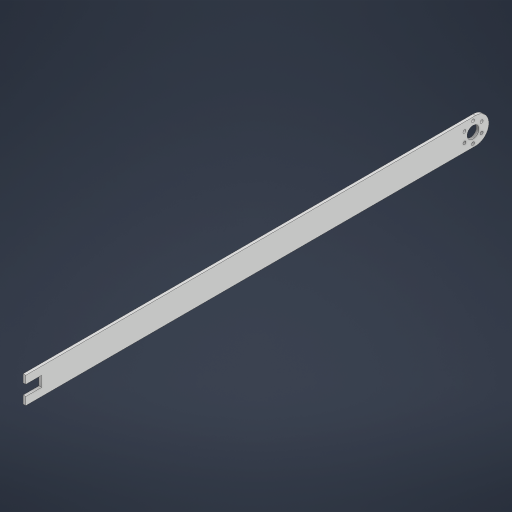
# Autodesk Inventor part: Arm
Saved by Autodesk Inventor 2023 (Build 270158000, 158)
## iProperties
Created: 2023-01-21
Part Number: Arm
Material: Generic
Document SubType Name: Modeling
Designer: Terrence
Density: 1 g/cm^3
Appearance: Default
Author: Terrence
Autodesk Inventor part; units mm, degrees
ref_plane "YZ Plane" through (0, 0, 0) normal (1, 0, 0) x (0, 1, 0)
ref_plane "XZ Plane" through (0, 0, 0) normal (0, 1, 0) x (-1, 0, 0)
ref_plane "XY Plane" through (0, 0, 0) normal (0, 0, 1) x (1, 0, 0)
sketch "Sketch1" plane through (0, 0, 0) normal (1, 0, 0) x (0, 1, 0)
  line L0 (0, -76.2) -> (63.5, -76.2)
  line L1 (63.5, -76.2) -> (63.5, -1193.8)
  line L2 (63.5, -1193.8) -> (0, -1193.8)
  line L3 (0, -1193.8) -> (0, -76.2)
  dimension "d0" = 63.5
  dimension "d1" = 1117.6
  constraints: 8 end point, 2 parallel, 1 horizontal, 1 perpendicular, 1 other
  measures "d0" distance of L1.end L2.end
  measures "d1" distance of L0.end L1.end
extrude "Extrusion1" add sketch "Sketch1" along normal blind 6.35
sketch "Sketch2" plane through (6.35, 0, 0) normal (1, 0, 0) x (0, 0, -1)
  line L0 (1193.8, 63.5) -> (76.2, 63.5) projected
  line L1 (1155.7, 63.5) -> (1155.7, 0) construction
  line L2 (0, 0) -> (1193.8, 0) projected
  circle A0 centre (1155.7, 31.75) radius 14.2875
  dimension "d5" = 1155.7
  dimension "d24" = 28.575
  constraints: 2 end point, 2 point on line, 1 centre point, 1 midpoint, 1 perpendicular
  measures "d5" distance from line of L2.start L1
  measures "d24" diameter of A0
extrude "Extrusion2" cut sketch "Sketch2" against normal through all
fillet "Fillet1" radius 31.75 2 edges at (3.175, 63.5, -1193.8) (3.175, 0, -1193.8)
sketch "Sketch5" plane through (6.35, 0, 0) normal (1, 0, 0) x (0, 0, -1)
  circle A0 centre (1155.7, 31.75) radius 14.2875 projected
  line L0 (1155.7, 31.75) -> (1155.7, 55.5752) construction
  circle A1 centre (1155.7, 55.5752) radius 3.6233
  point P0 (0, 0)
  dimension "d32" = 23.8252
  constraints: 2 end point, 1 centre point, 1 coincident, 1 vertical
  measures "d32" distance of L0.start L0.end
extrude "Extrusion5" cut sketch "Sketch5" against normal through all contours A1
pattern_circular "Circular Pattern1" count 6 over 360 about axis through (6.35, 31.75, -1155.7) along (-1, 0, 0) of "Extrusion5"
sketch "Sketch8" plane through (6.35, 0, 0) normal (1, 0, 0) x (0, 0, -1)
  line L0 (76.2, 44.45) -> (114.3, 44.45)
  line L1 (114.3, 44.45) -> (114.3, 19.05)
  line L2 (114.3, 19.05) -> (76.2, 19.05)
  line L3 (76.2, 19.05) -> (76.2, 44.45)
  line L4 (76.2, 63.5) -> (76.2, 0) projected
  point P0 (0, 0)
  point P1 (76.2, 31.75)
  dimension "d44" = 38.1
  dimension "d45" = 25.4
  constraints: 8 end point, 2 midpoint, 2 parallel, 1 horizontal, 1 perpendicular
  measures "d44" distance of L1.end L2.end
  measures "d45" distance of L2.end L0.start
extrude "Extrusion8" cut sketch "Sketch8" against normal blind 25.4
body "Solid1"
